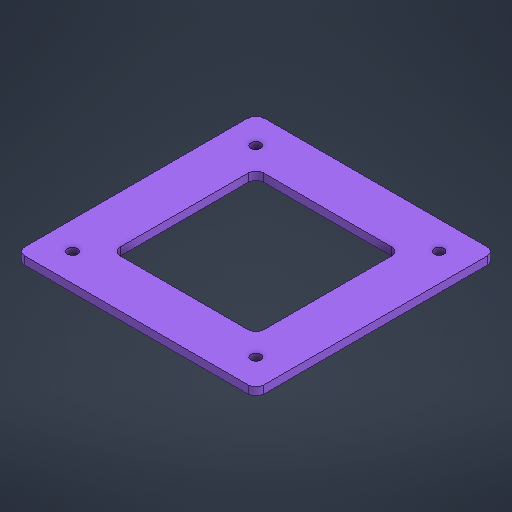
# Autodesk Inventor part: top
Saved by Autodesk Inventor 2026 (Build 300175000, 175)
## iProperties
Created: 2025-04-15
Part Number: top
Material: Generic
Document SubType Name: Modeling
Designer: ADM
Density: 1 g/cm^3
Appearance: Violet
Author: ADM
Autodesk Inventor part; units mm, degrees
ref_plane "YZ Plane" through (0, 0, 0) normal (1, 0, 0) x (0, 1, 0)
ref_plane "XZ Plane" through (0, 0, 0) normal (0, 1, 0) x (-1, 0, 0)
ref_plane "XY Plane" through (0, 0, 0) normal (0, 0, 1) x (1, 0, 0)
sketch "Sketch2" plane through (0, 0, 0) normal (0, 1, 0) x (-1, 0, 0)
  line L0 (2, 0) -> (58, 0)
  line L1 (60, -2) -> (60, -58)
  line L2 (58, -60) -> (2, -60)
  line L3 (0, -58) -> (0, -2)
  line L4 (48, -46) -> (48, -14)
  line L5 (46, -12) -> (14, -12)
  line L6 (12, -14) -> (12, -46)
  line L7 (14, -48) -> (46, -48)
  arc A0 (60, -2) -> (58, 0) centre (58, -2) ccw
  arc A1 (58, -60) -> (60, -58) centre (58, -58) ccw
  arc A2 (0, -58) -> (2, -60) centre (2, -58) ccw
  arc A3 (2, 0) -> (0, -2) centre (2, -2) ccw
  arc A4 (14, -12) -> (12, -14) centre (14, -14) ccw
  arc A5 (12, -46) -> (14, -48) centre (14, -46) ccw
  arc A6 (46, -48) -> (48, -46) centre (46, -46) ccw
  arc A7 (48, -14) -> (46, -12) centre (46, -14) ccw
  point P0 (0, 0)
  point P1 (60, -60)
  point P2 (60, 0)
  point P3 (0, -60)
  dimension "d9" = 60
  dimension "d10" = 60
  dimension "d11" = 12
  dimension "d12" = 2
  constraints: 16 end point, 16 point on circle, 16 tangent, 8 centre point, 8 point on line, 7 equal radius, 4 parallel, 2 perpendicular, 1 horizontal, 3 other
  measures "d9" distance of point (60, -60) point (0, -60)
  measures "d10" distance of point (60, 0) point (60, -60)
  measures "d11" distance between parallel lines of L1 L4
  measures "d12" radius of A0
extrude "Extrusion2" add sketch "Sketch2" along normal blind 2
sketch "Sketch4" plane through (0, 2, 0) normal (0, 1, 0) x (1, 0, 0)
  circle A0 centre (-53.0047, 6.9783) radius 1.25
  circle A1 centre (-53.0047, 52.9688) radius 1.25
  circle A2 centre (-7.0099, 6.9783) radius 1.25
  circle A3 centre (-7.0099, 52.9688) radius 1.25
  point P0 (0, 0)
  dimension "d27" = 2.5
  dimension "d28" = 2.5
  dimension "d29" = 2.5
  dimension "d30" = 2.5
  constraints: 4 centre point
  measures "d27" diameter of A0
  measures "d28" diameter of A1
  measures "d29" diameter of A2
  measures "d30" diameter of A3
extrude "Extrusion3" cut sketch "Sketch4" against normal through all
body "Solid2"
